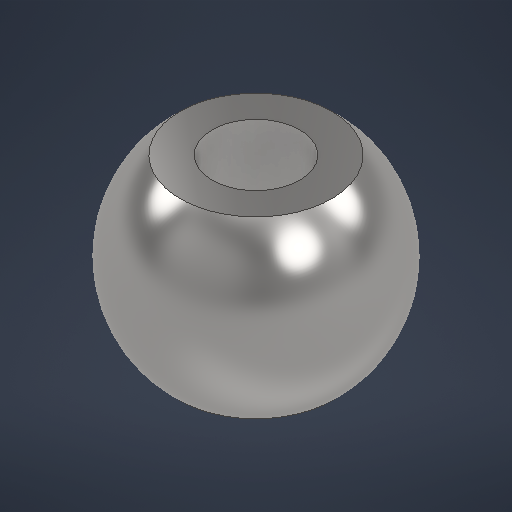
# Autodesk Inventor part: Ball
Saved by Autodesk Inventor 2025 (Build 290162000, 162)
## iProperties
Created: 2024-10-17
Part Number: Ball
Material: Нержавеющая сталь
Document SubType Name: Modeling
Designer: khrip
Density: 8 g/cm^3
Appearance: С умеренной полировкой
Author: khrip
Autodesk Inventor part; units mm, degrees
ref_plane "YZ Plane" through (0, 0, 0) normal (1, 0, 0) x (0, 1, 0)
ref_plane "XZ Plane" through (0, 0, 0) normal (0, 1, 0) x (-1, 0, 0)
ref_plane "XY Plane" through (0, 0, 0) normal (0, 0, 1) x (1, 0, 0)
sketch "Эскиз1" plane through (0, 0, 0) normal (0, 1, 0) x (-1, 0, 0)
  circle A0 centre (0, 0) radius 3.969
  line L0 (3.969, 0) -> (-3.969, 0)
  dimension "d0" = 7.938
  dimension "d1" = 7.938
  constraints: 2 end point, 2 point on circle, 1 centre point, 1 coincident, 1 horizontal
  measures "d0" diameter of A0
  measures "d1" distance of L0.start L0.end
revolve "Вращение1" add sketch "Эскиз1" angle 360 about axis through (-3.969, 0, 0) along (1, 0, 0) picked at (1.323, -1.2297) contours A0 L0
sketch "Эскиз2" plane through (0, 0, 0) normal (0, 1, 0) x (-1, 0, 0)
  circle A0 centre (0, 0) radius 1.5
  dimension "d3" = 3
  constraints: 1 centre point, 1 coincident
  measures "d3" diameter of A0
extrude "Выдавливание1" cut sketch "Эскиз2" along normal mid plane 10
sketch "Эскиз3" plane through (0, 0, 0) normal (1, 0, 0) x (0, 1, 0)
  line L0 (13, 10) -> (3, 10)
  line L1 (3, 10) -> (3, -10)
  line L2 (3, -10) -> (13, -10)
  line L3 (13, -10) -> (13, 10)
  point P0 (0, 0)
  dimension "d6" = 3
  dimension "d7" = 20
  dimension "d8" = 10
  dimension "d9" = 10
  constraints: 8 end point, 2 parallel, 1 horizontal, 1 perpendicular
  measures "d6" distance from line of L1 point (0, 0)
  measures "d7" distance between parallel lines of L2 L0
  measures "d8" distance between parallel lines of L1 L3
  measures "d9" distance from line of point (0, 0) L0
extrude "Выдавливание2" cut sketch "Эскиз3" along normal through all both and the other way through all
mirror "Зеркальное отражение1" about plane through (0, 0, 0) normal (0, 1, 0) of "Выдавливание2"
